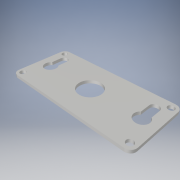
# Autodesk Inventor part: Back Plate
Saved by Autodesk Inventor 2019 (Build 230136000, 136)
## iProperties
Created: 2019-03-05
Part Number: Back Plate
Material: Aluminum 6061
Document SubType Name: Modeling
Designer: Jackson Smith
Density: 2.7 g/cm^3
Appearance: Aluminum - Flat
Author: Jackson Smith
Autodesk Inventor part; units mm, degrees
ref_plane "YZ Plane" through (0, 0, 0) normal (1, 0, 0) x (0, 1, 0)
ref_plane "XZ Plane" through (0, 0, 0) normal (0, 1, 0) x (-1, 0, 0)
ref_plane "XY Plane" through (0, 0, 0) normal (0, 0, 1) x (1, 0, 0)
sketch "Sketch1" plane through (0, 0, 0) normal (0, 1, 0) x (-1, 0, 0)
  line L0 (-32.5, -15) -> (32.5, -15)
  line L1 (32.5, -15) -> (32.5, 15)
  line L2 (32.5, 15) -> (-32.5, 15)
  line L3 (-32.5, 15) -> (-32.5, -15)
  line L4 (-32.5, -15) -> (32.5, 15) construction
  line L5 (32.5, -15) -> (-32.5, 15) construction
  point P0 (0, 0)
  dimension "d0" = 65
  dimension "d1" = 30
  constraints: 12 end point, 2 midpoint, 2 parallel, 1 horizontal, 1 perpendicular
  measures "d0" distance of L2.end L1.end
  measures "d1" distance of L1.end L0.end
extrude "Extrusion1" add sketch "Sketch1" along normal blind 1.5875
fillet "Fillet1" radius 3 4 edges at (-32.5, 0.7937, -15) (-32.5, 0.7937, 15) (32.5, 0.7937, 15) (32.5, 0.7937, -15)
sketch "Sketch2" plane through (0, 1.5875, 0) normal (0, 1, 0) x (1, 0, 0)
  point P0 (0, 0)
hole "Hole1" at (0, 1.5875, 0) direction (0, -1, 0) diameter 12 end through all
sketch "Sketch3" plane through (0, 1.5875, 0) normal (0, 1, 0) x (1, 0, 0)
  arc A0 (-27.5, 2.681) -> (-23, 2.681) centre (-25.25, 0) ccw
  line L0 (-27.5, 2.681) -> (-27.5, 7.78)
  line L1 (-23, 7.78) -> (-23, 2.681)
  arc A1 (-25.25, 10.03) -> (-27.5, 7.78) centre (-25.25, 7.78) ccw
  arc A2 (-23, 7.78) -> (-25.25, 10.03) centre (-25.25, 7.78) ccw
  point P0 (0, 0)
  point P1 (-25.25, 10.03)
  dimension "d12" = 7
  dimension "d15" = 4.5
  dimension "d16" = 2.25
  dimension "d17" = 10.03
  dimension "d18" = 25.25
  constraints: 6 point on circle, 4 end point, 3 centre point, 2 tangent, 2 vertical, 1 concentric, 1 horizontal alignment, 1 vertical alignment, 6 other
  measures "d12" diameter of A0
  measures "d15" distance between parallel lines of L1 L0
  measures "d16" radius of A1
  measures "d17" distance of A0.centre point (-25.25, 10.03)
  measures "d18" distance of point (0, 0) A0.centre
extrude "Extrusion2" cut sketch "Sketch3" against normal through all
mirror "Mirror1" about plane through (0, 0, 0) normal (1, 0, 0) of "Extrusion2"
sketch "Sketch4" plane through (0, 1.5875, 0) normal (0, 1, 0) x (1, 0, 0)
  arc A0 (-29.5, 15) -> (-32.5, 12) centre (-29.5, 12) ccw projected
  arc A1 (-32.5, -12) -> (-29.5, -15) centre (-29.5, -12) ccw projected
  arc A2 (29.5, -15) -> (32.5, -12) centre (29.5, -12) ccw projected
  arc A3 (32.5, 12) -> (29.5, 15) centre (29.5, 12) ccw projected
  point P0 (0, 0)
  constraints: 4 coincident
hole "Hole2" at (-29.5, 1.5875, -12) at (-29.5, 1.5875, 12) at (29.5, 1.5875, 12) at (29.5, 1.5875, -12) direction (0, -1, 0) diameter 3.175 end through all
body "Solid1"
